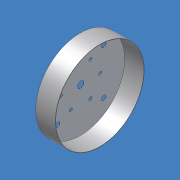
# Autodesk Inventor part: bottom cap
Saved by Autodesk Inventor 2015 (Build 190159000, 159)
## iProperties
Created: 2005-07-05
Part Number: bottom cap
Document SubType Name: Modeling
Designer: jony
Material: Generic
Density: 1 g/cm^3
Appearance: Default
Author: jony
Autodesk Inventor part; units mm, degrees
ref_plane "YZ Plane" through (0, 0, 0) normal (1, 0, 0) x (0, 1, 0)
ref_plane "XZ Plane" through (0, 0, 0) normal (0, 1, 0) x (-1, 0, 0)
ref_plane "XY Plane" through (0, 0, 0) normal (0, 0, 1) x (1, 0, 0)
sketch "Sketch1" plane through (0, 0, 0) normal (1, 0, 0) x (0, 1, 0)
  circle A0 centre (0, 0) radius 86.5188
  circle A1 centre (0, 0) radius 6.35
  circle A2 centre (-38.1, 0) radius 3.175
  circle A3 centre (-19.05, -32.9956) radius 3.175
  circle A4 centre (19.05, -32.9956) radius 3.175
  circle A5 centre (38.1, 0) radius 3.175
  circle A6 centre (19.05, 32.9956) radius 3.175
  circle A7 centre (-19.05, 32.9956) radius 3.175
  circle A8 centre (-44.9072, -44.9072) radius 4.7625
  line L0 (0, 0) -> (-44.9072, -44.9072) construction
  line L1 (0, 0) -> (0, -86.5188) construction
  circle A9 centre (44.9072, -44.9072) radius 4.7625
  circle A10 centre (44.9072, 44.9072) radius 4.7625
  circle A11 centre (-44.9072, 44.9072) radius 4.7625
  dimension "d0" = 173.0375
  dimension "d1" = 12.7
  dimension "d2" = 6.35
  dimension "d3" = 38.1
  dimension "d6" = 360
  dimension "d8" = 9.525
  dimension "d9" = 45
  dimension "d13" = 360
  dimension "d26" = 89.8144
  constraints: 11 centre point, 4 end point, 2 coincident, 1 horizontal alignment, 1 vertical, 1 vertical alignment, 24 other
  measures "d1" diameter of A1
  measures "d2" diameter of A2
  measures "d3" distance of point (0, 0) A2.centre
  measures "d8" diameter of A8
  measures "d9" angle of L1 L0
  measures "d26" distance of A9.centre L0.end
extrude "Extrusion1" add sketch "Sketch1" along normal blind 38.1
hole "Hole1" at (38.1, 0, 0) direction (-1, 0, 0) diameter 171.45 depth 37.3062
body "Solid1"
